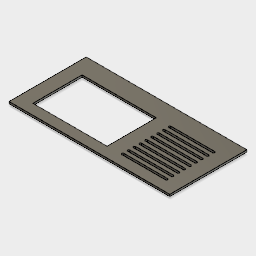
charlesBox_top (Autodesk Fusion 360 design; units mm, degrees)
Autodesk Fusion 360 part; units mm, degrees
sketch "Sketch1" plane through (0, 0, 0) normal (0, 1, 0) x (1, 0, 0)
  line L0 (77, 37) -> (-77, 37)
  line L1 (-77, 37) -> (-77, -37)
  line L2 (-77, -37) -> (77, -37)
  line L3 (77, -37) -> (77, 37)
  line L4 (77, 37) -> (-77, -37) construction
  line L5 (-77, 37) -> (77, -37) construction
  line L6 (7, 20) -> (-64, 20)
  line L7 (-64, 20) -> (-64, -27)
  line L8 (-64, -27) -> (7, -27)
  line L9 (7, -27) -> (7, 20)
  point P0 (-6.9256, 0)
  dimension "d1" = 74
  dimension "d2" = 154
  dimension "d3" = 70
  dimension "d4" = 17
  dimension "d5" = 10
  dimension "d6" = 13
  measures "d1" distance of L0.start L2.end
  measures "d2" distance of L0.start L0.end
  measures "d3" distance of L3 L9
  measures "d4" distance of L0 L6
  measures "d5" distance of L2 L8
  measures "d6" distance of L1 L7
extrude "Extrude1" add sketch "Sketch1" along normal blind 2
sketch "Sketch2" plane through (0, 0, 0) normal (0, -1, 0) x (1, 0, 0)
  line L0 (77, -37) -> (77, 37)
  line L1 (77, 37) -> (-77, 37)
  line L2 (-77, 37) -> (-77, -37)
  line L3 (-77, -37) -> (77, -37)
  line L4 (77, 37) -> (77, -37)
  line L5 (77, -37) -> (-77, -37)
  line L6 (-77, -37) -> (-77, 37)
  line L7 (-77, 37) -> (77, 37)
  line L8 (75, 35) -> (-75, 35)
  line L9 (-75, 35) -> (-75, -35)
  line L10 (-75, -35) -> (75, -35)
  line L11 (75, -35) -> (75, 35)
  line L12 (75, 35) -> (-75, -35) construction
  line L13 (-75, 35) -> (75, -35) construction
  line L14 (73, 33) -> (-73, 33)
  line L15 (-73, 33) -> (-73, -33)
  line L16 (-73, -33) -> (73, -33)
  line L17 (73, -33) -> (73, 33)
  line L18 (73, 33) -> (-73, -33) construction
  line L19 (-73, 33) -> (73, -33) construction
  dimension "d9" = 2
  dimension "d10" = 2
  dimension "d11" = 2
  dimension "d12" = 2
  measures "d9" distance of L0 L11
  measures "d10" distance of L1 L8
  measures "d11" distance of L8 L14
  measures "d12" distance of L9 L15
extrude "Extrude2" add sketch "Sketch2" along normal blind 2 contours L8 L9 L10 L11
sketch "Sketch3" plane through (0, 0, 0) normal (0, 1, 0) x (1, 0, 0)
  line L0 (20, 18) -> (64, 18)
  line L1 (64, 18) -> (64, 20)
  line L2 (64, 20) -> (20, 20)
  line L3 (20, 20) -> (20, 18)
  line L4 (77, -37) -> (77, 37)
  line L5 (7, 20) -> (7, -27)
  dimension "d15" = 2
  dimension "d16" = 13
  dimension "d17" = 13
  measures "d15" distance of L0.start L2.end
  measures "d16" distance of L1.end L4
  measures "d17" distance of L3 L5
extrude "Extrude3" cut sketch "Sketch3" along normal up to surface (2 mm away)
fillet "Fillet1" radius 1 4 edges at (20, 1, -20) (20, 1, -18) (64, 1, -20) (64, 1, -18)
pattern_linear "R-Pattern1" count 9 spacing 5.625 along (0, 0, 1) of "Extrude3", "Fillet1"
equation "d10 = d9"
equation "d11 = d9"
equation "d12 = d10"
